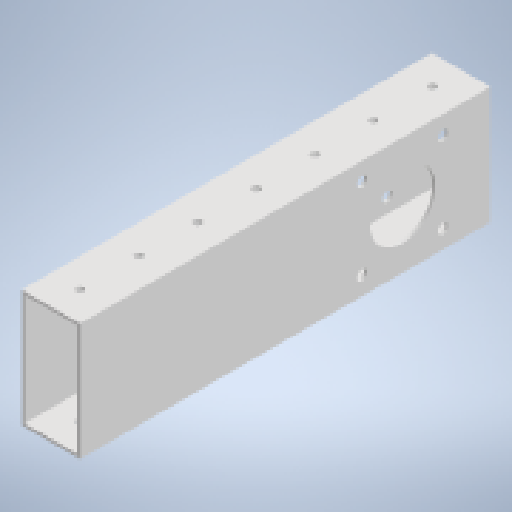
# Autodesk Inventor part: VersaFrame (Jumper Bar)
Saved by Autodesk Inventor 2023 (Build 270158000, 158)
## iProperties
Created: 2020-01-13
Part Number: VersaFrame (Jumper Bar)
Material: Generic
Document SubType Name: Modeling
Designer: aidan
Density: 1 g/cm^3
Appearance: Default
Author: aidan
Autodesk Inventor part; units mm, degrees
ref_plane "YZ Plane" through (0, 0, 0) normal (1, 0, 0) x (0, 1, 0)
ref_plane "XZ Plane" through (0, 0, 0) normal (0, 1, 0) x (-1, 0, 0)
ref_plane "XY Plane" through (0, 0, 0) normal (0, 0, 1) x (1, 0, 0)
sketch "Sketch1" plane through (0, 0, 0) normal (0, 0, 1) x (1, 0, 0)
  line L0 (-12.1708, 16.0073) -> (13.2292, 16.0073)
  line L1 (13.2292, 16.0073) -> (13.2292, -34.7927)
  line L2 (13.2292, -34.7927) -> (-12.1708, -34.7927)
  line L3 (-12.1708, -34.7927) -> (-12.1708, 16.0073)
  line L4 (11.9592, 14.7373) -> (-10.9008, 14.7373)
  line L5 (-10.9008, 14.7373) -> (-10.9008, -33.5227)
  line L6 (-10.9008, -33.5227) -> (11.9592, -33.5227)
  line L7 (11.9592, -33.5227) -> (11.9592, 14.7373)
  point P0 (0, 0)
  dimension "d0" = 25.4
  dimension "d1" = 50.8
  dimension "d2" = 1.27
  constraints: 16 end point, 4 parallel, 2 perpendicular, 1 horizontal, 3 other
  measures "d0" distance of L0.start L0.end
  measures "d1" distance of L0.end L1.end
  measures "d2" distance between parallel lines of L0 L4
extrude "Extrusion1" add sketch "Sketch1" along normal blind 177.8
sketch "Sketch2" plane through (-12.1708, 16.0073, 0) normal (0, 1, 0) x (1, 0, 0)
  circle A0 centre (12.7, -12.7) radius 1.7272
  line L0 (25.4, 0) -> (0, 0) projected
  line L1 (0, 0) -> (0, -177.8) projected
  point P0 (12.1708, 0)
  dimension "d5" = 3.4544
  dimension "d6" = 12.7
  dimension "d7" = 12.7
  constraints: 1 centre point
  measures "d5" diameter of A0
  measures "d6" distance from line of L0 A0.centre
  measures "d7" distance from line of L1 A0.centre
extrude "Extrusion2" cut sketch "Sketch2" against normal through all
pattern_linear "Rectangular Pattern1" count 18 spacing 25.4 along (0, 0, 1) of "Extrusion2"
sketch "Sketch3" plane through (13.2292, -34.7927, 0) normal (1, 0, 0) x (0, 0, -1)
  circle A0 centre (-38.1, 25.4) radius 14.2875
  line L0 (0, 0) -> (-177.8, 0) projected
  line L1 (0, 0) -> (0, 50.8) projected
  circle A1 centre (-38.1, 25.4) radius 24.7523
  line L2 (-20.5975, 42.9025) -> (-55.6025, 42.9025)
  line L3 (-55.6025, 42.9025) -> (-55.6025, 7.8975)
  line L4 (-55.6025, 7.8975) -> (-20.5975, 7.8975)
  line L5 (-20.5975, 7.8975) -> (-20.5975, 42.9025)
  circle A2 centre (-20.5975, 42.9025) radius 2.159
  circle A3 centre (-20.5975, 7.8975) radius 2.159
  circle A4 centre (-55.6025, 7.8975) radius 2.159
  circle A5 centre (-55.6025, 42.9025) radius 2.159
  point P0 (0, 34.7927)
  point P1 (0, 25.4)
  dimension "d15" = 28.575
  dimension "d16" = 25.4
  dimension "d17" = 38.1
  dimension "d20" = 49.5046
  dimension "d22" = 4.318
  dimension "d23" = 4.318
  dimension "d24" = 4.318
  dimension "d25" = 4.318
  constraints: 8 end point, 6 centre point, 5 coincident, 3 point on circle, 2 parallel, 2 perpendicular, 1 horizontal, 1 midpoint
  measures "d15" diameter of A0
  measures "d16" distance from line of L0 A0.centre
  measures "d17" distance of point (0, 25.4) A0.centre
  measures "d20" diameter of A1
  measures "d22" diameter of A2
  measures "d23" diameter of A3
  measures "d24" diameter of A4
  measures "d25" diameter of A5
extrude "Extrusion3" cut sketch "Sketch3" against normal blind 25.4 contours A0 | A2 L5 A1 | A1 A2 | A3 A1 | A1 L5 A3 | L2 A2 A1 | L5 A2 L2 | A1 A3 L4 | L4 A3 L5 | A5 L2 A1 | A1 A5 | A5 L3 L2 | A4 A1 | A1 L4 A4 | L4 L3 A4 | L3 A5 A1 | A1 A4 L3
equation "\"d3\" = d13"
equation "\"d23\" = d22"
equation "\"d24\" = d22"
equation "\"d25\" = d22"
equation "\"d10\" = d14"
equation "\"d13\" = 177.8"
equation "\"d14\" = d13"
body "Solid1"
